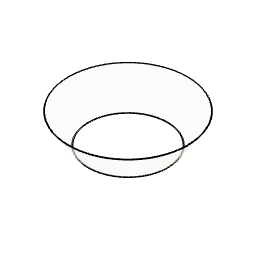
jalkalampunvarjostin v3 (Autodesk Fusion 360 design; units mm, degrees)
Autodesk Fusion 360 part; units mm, degrees
sketch "Sketch1" plane through (0, 0, 0) normal (0, 1, 0) x (1, 0, 0)
  line L0 (0, 0) -> (0, -75) construction
  line L1 (0, -75) -> (150, -75) construction
  line L2 (0, 0) -> (99, 0) construction
  line L3 (99, 0) -> (150, -75)
  line L4 (150, -75) -> (152, -75)
  line L5 (99, 0) -> (101, 0)
  line L6 (101, 0) -> (152, -75)
  dimension "d2" = 75
  dimension "d3" = 150
  dimension "d12" = 99
  dimension "d13" = 2
  dimension "d14" = 2
  constraint coincident L0.start L2.start
  constraint perpendicular L0 L1
  constraint perpendicular L0 L2
  constraint parallel L1 L4
  constraint parallel L2 L5
  measures "d2" distance of L0.start L0.end
  measures "d3" distance of L0.end L1.end
  measures "d12" distance of L0.start L2.end
  measures "d13" distance of L1.end L4.end
  measures "d14" distance of L2.end L5.end
revolve "Revolve2" add sketch "Sketch1" angle 360 about axis through (0, 0, 0) along (0, 0, 1)
fillet "Fillet2" radius 0.5 1 edges at (-141.7138, -54.9655, 75)
equation "d3 = ( 300 / 2 ) * 1 mm"
equation "d12 = ( 198 / 2 ) * 1 mm"
equation "d13 = materialthickness"
equation "d14 = materialthickness"
equation "materialthickness = 2 mm"
